Head Motor (Autodesk Fusion 360 design; units mm, degrees)
Autodesk Fusion 360 part; units mm, degrees
note: some values were not read from the file. Set by a fixed rule: which sketch regions a step uses.
sketch "Sketch1" plane through (0, 0, 0) normal (0, 0, 1) x (1, 0, 0)
  line L0 (-16, -23) -> (16, -23)
  line L1 (16, -23) -> (16, 23)
  line L2 (16, 23) -> (-16, 23)
  line L3 (-16, 23) -> (-16, -23)
  line L4 (-16, -23) -> (16, 23) construction
  line L5 (16, -23) -> (-16, 23) construction
  dimension "d1" = 46
  dimension "d2" = 32
  constraint perpendicular L0 L1
  constraint parallel L0 L2
  constraint parallel L1 L3
  constraint horizontal L0
  constraint coincident L4 origin
  constraint coincident L5 origin
  measures "d1" distance of L0.end L1.end
  measures "d2" distance of L1.end L2.end
extrude "Extrude1" add sketch "Sketch1" along normal blind 23
sketch "Sketch2" plane through (0, 0, 23) normal (0, 0, 1) x (-1, 0, 0)
  line L0 (16, -23) -> (16, 23)
  line L1 (16, 23) -> (-16, 23)
  line L2 (-16, 23) -> (-16, -23)
  line L3 (-16, -23) -> (16, -23)
  line L4 (-9, 16.5) -> (9, 16.5) construction
  line L5 (9, 16.5) -> (9, -16.5) construction
  line L6 (9, -16.5) -> (-9, -16.5) construction
  line L7 (-9, -16.5) -> (-9, 16.5) construction
  line L8 (-9, 16.5) -> (9, -16.5) construction
  line L9 (9, 16.5) -> (-9, -16.5) construction
  circle A0 centre (-9, -16.5) radius 3.5
  circle A1 centre (9, -16.5) radius 3.5
  circle A2 centre (-9, 16.5) radius 3.5
  circle A3 centre (9, 16.5) radius 3.5
  line L10 (0, -23) -> (0, 23) construction
  circle A4 centre (0, -8) radius 3
  circle A5 centre (9, -16.5) radius 1.5
  circle A6 centre (-9, -16.5) radius 1.5
  circle A7 centre (9, 16.5) radius 1.5
  circle A8 centre (-9, 16.5) radius 1.5
  dimension "d5" = 33
  dimension "d6" = 18
  dimension "d7" = 7
  dimension "d8" = 7
  dimension "d9" = 7
  dimension "d10" = 7
  dimension "d13" = 6
  dimension "d14" = 15
  dimension "d34" = 3
  dimension "d35" = 3
  dimension "d36" = 3
  dimension "d37" = 3
  constraint perpendicular L4 L5
  constraint parallel L4 L6
  constraint parallel L5 L7
  constraint horizontal L4
  constraint coincident L8 origin
  constraint coincident L9 origin
  constraint coincident L6.end L7.start
  constraint coincident L5.end L6.start
  constraint coincident L4.start L7.end
  constraint coincident L4.end L5.start
  constraint midpoint L3 L10.start
  constraint midpoint L1 L10.end
  constraint coincident L10 A4.centre
  constraint concentric A1 A5
  constraint concentric A3 A7
  constraint concentric A2 A8
  measures "d5" distance of L4.end L5.end
  measures "d6" distance of L5.end L6.end
  measures "d7" diameter of A0
  measures "d8" diameter of A1
  measures "d9" diameter of A2
  measures "d10" diameter of A3
  measures "d13" diameter of A4
  measures "d14" distance of L3 A4.centre
  measures "d34" diameter of A5
  measures "d35" diameter of A6
  measures "d36" diameter of A7
  measures "d37" diameter of A8
extrude "Extrude2" add sketch "Sketch2" along normal blind 2 contours A0 | A1 | A2 | A3
extrude "Extrude3" add sketch "Sketch2" along normal blind 19 contours A4
fillet "Fillet1" radius 1 4 faces at (16, -7.6667, 7.6667) (-5.3333, -23, 7.6667) (-16, 7.6667, 7.6667) (5.3333, 23, 7.6667)
fillet "Fillet2" radius 0.5 1 edges at (-5.7369, -15.2343, 25) 4 faces at (6.1853, 16.7484, 25) (6.1853, -16.2516, 25) (-11.8147, 16.7484, 25) (-11.8147, -16.2516, 25)
fillet "Fillet3" radius 1 1 faces at (0.5, 8.866, 42)
sketch "Sketch4" plane through (-3, 23, 11.5) normal (0, 1, 0) x (-1, 0, 0)
sketch "Sketch5" plane through (0, -23, 0) normal (0, -1, 0) x (1, 0, 0)
  line L0 (-15, 1) -> (15, 1)
  line L1 (15, 1) -> (15, 22)
  line L2 (15, 22) -> (-15, 22)
  line L3 (-15, 22) -> (-15, 1)
  circle A0 centre (3, 10) radius 12
  point P0 (16, 22)
  dimension "d25" = 24
  dimension "d26" = 10
  dimension "d27" = 13
  measures "d25" diameter of A0
  measures "d26" vertical distance of origin A0.centre
  measures "d27" horizontal distance of A0.centre P0
extrude "Extrude5" add sketch "Sketch5" along normal blind 31 contours L0 A0 | L0 A0
sketch "Sketch8" plane through (0, -54, 0) normal (0, -1, 0) x (1, 0, 0)
  circle A0 centre (3, 10) radius 12
  circle A1 centre (3, 10) radius 11.8
  dimension "d31" = -0.2
extrude "Extrude6" cut sketch "Sketch8" against normal blind 1 contours A1
